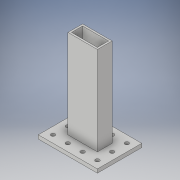
# Autodesk Inventor part: PostForHexAxel
Saved by Autodesk Inventor 2017 (Build 210142000, 142)
## iProperties
Created: 2016-05-18
Part Number: PostForHexAxel
Material: Generic
Document SubType Name: Modeling
Designer: steele
Density: 1 g/cm^3
Appearance: Default
Author: steele
Autodesk Inventor part; units mm, degrees
ref_plane "YZ Plane" through (0, 0, 0) normal (1, 0, 0) x (0, 1, 0)
ref_plane "XZ Plane" through (0, 0, 0) normal (0, 1, 0) x (-1, 0, 0)
ref_plane "XY Plane" through (0, 0, 0) normal (0, 0, 1) x (1, 0, 0)
sketch "Sketch1" plane through (0, 0, 0) normal (0, 1, 0) x (-1, 0, 0)
  line L0 (50.8, 38.1) -> (-50.8, 38.1)
  line L1 (-50.8, 38.1) -> (-50.8, -38.1)
  line L2 (-50.8, -38.1) -> (50.8, -38.1)
  line L3 (50.8, -38.1) -> (50.8, 38.1)
  line L4 (50.8, 38.1) -> (-50.8, -38.1) construction
  line L5 (-50.8, 38.1) -> (50.8, -38.1) construction
  point P0 (0, 0)
  dimension "d0" = 76.2
  dimension "d1" = 101.6
  constraints: 12 end point, 2 midpoint, 2 parallel, 1 horizontal, 1 perpendicular
  measures "d0" distance of L0.end L1.end
  measures "d1" distance of L0.start L0.end
extrude "Extrusion1" add sketch "Sketch1" along normal blind 6.35
sketch "Sketch2" plane through (0, 6.35, 0) normal (0, 1, 0) x (1, 0, 0)
  line L0 (25.4, -12.7) -> (25.4, 12.7)
  line L1 (25.4, 12.7) -> (-25.4, 12.7)
  line L2 (-25.4, 12.7) -> (-25.4, -12.7)
  line L3 (-25.4, -12.7) -> (25.4, -12.7)
  line L4 (25.4, -12.7) -> (-25.4, 12.7) construction
  line L5 (25.4, 12.7) -> (-25.4, -12.7) construction
  line L6 (22.225, -9.525) -> (22.225, 9.525)
  line L7 (22.225, 9.525) -> (-22.225, 9.525)
  line L8 (-22.225, 9.525) -> (-22.225, -9.525)
  line L9 (-22.225, -9.525) -> (22.225, -9.525)
  line L10 (22.225, -9.525) -> (-22.225, 9.525) construction
  line L11 (22.225, 9.525) -> (-22.225, -9.525) construction
  point P0 (0, 0)
  dimension "d4" = 50.8
  dimension "d5" = 25.4
  dimension "d6" = 3.175
  dimension "d7" = 3.175
  constraints: 24 end point, 4 midpoint, 4 parallel, 2 perpendicular, 2 vertical
  measures "d4" distance of L2.end L0.start
  measures "d5" distance of L1.end L2.end
  measures "d6" distance between parallel lines of L3 L9
  measures "d7" distance between parallel lines of L0 L6
extrude "Extrusion2" add sketch "Sketch2" along normal blind 152.4
sketch "Sketch5" plane through (0, 6.35, 0) normal (0, 1, 0) x (1, 0, 0)
  line L0 (-51.0645, -25.4) -> (50.8, -25.4) construction
  line L1 (50.8, -38.1) -> (50.8, 38.1) construction
  line L2 (-38.1, -38.1) -> (-38.1, 38.1) construction
  line L3 (50.8, 38.1) -> (-50.8, 38.1) construction
  line L4 (-50.8, -38.1) -> (50.8, -38.1) construction
  line L5 (-50.8, 38.1) -> (-50.8, -38.1) construction
  point P0 (0, 0)
  point P1 (-38.1, -25.4)
  point P2 (-12.7, -25.4)
  point P3 (12.7, -25.4)
  point P4 (38.1, -25.4)
  point P5 (-38.1, 0)
  point P6 (-12.7, 0)
  point P7 (12.7, 0)
  point P8 (38.1, 0)
  point P9 (-38.1, 25.4)
  point P10 (-12.7, 25.4)
  point P11 (12.7, 25.4)
  point P12 (38.1, 25.4)
  dimension "d19" = 12.7
  dimension "d20" = 12.7
  dimension "d23" = 25.4
  dimension "d26" = 25.4
  constraints: 4 end point, 4 point on line, 2 horizontal, 1 perpendicular, 1 vertical, 11 other
  measures "d19" distance between parallel lines of L4 L0
  measures "d20" distance between parallel lines of L5 L2
  measures "d23" distance of point (-38.1, -25.4) point (-12.7, -25.4)
  measures "d26" distance of point (-38.1, -25.4) point (-38.1, 0)
hole "Hole2" at (-38.1, 6.35, 25.4) at (-12.7, 6.35, 25.4) at (12.7, 6.35, 25.4) at (38.1, 6.35, 25.4) at (-38.1, 6.35, 0) at (-12.7, 6.35, 0) at (12.7, 6.35, 0) at (38.1, 6.35, 0) at (-38.1, 6.35, -25.4) at (-12.7, 6.35, -25.4) at (12.7, 6.35, -25.4) at (38.1, 6.35, -25.4) direction (0, -1, 0) diameter 6.7564 end through all clearance for "Flat Head Machine Screw (82)" size "1/4" standard "Ansi Unified Screw Threads"
body "Solid1"
